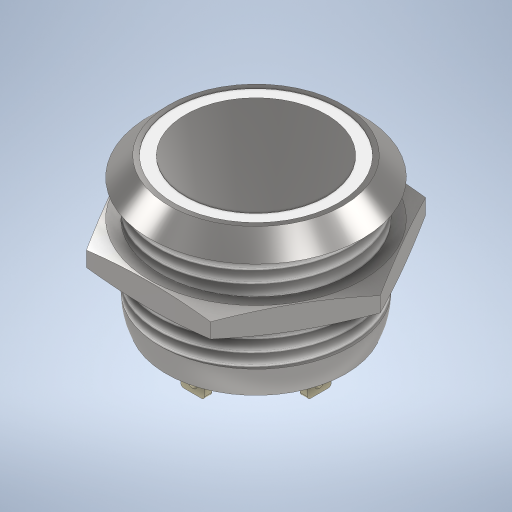
# Autodesk Inventor part: 16mm LED Pushbutton
Saved by Autodesk Inventor 2024 (Build 280153000, 153)
## iProperties
Created: 2024-08-19
Part Number: 16mm LED Pushbutton
Material: Stainless Steel
Document SubType Name: Modeling
Designer: Ishaan
Density: 8 g/cm^3
Appearance: Semi-Polished
Author: Ishaan
Autodesk Inventor part; units mm, degrees
ref_plane "YZ Plane" through (0, 0, 0) normal (1, 0, 0) x (0, 1, 0)
sketch "Sketch1" plane through (0, 0, 0) normal (0, 0, 1) x (1, 0, 0)
  line L0 (0, 11.85) -> (7.3, 11.85)
  line L1 (7.3, 11.85) -> (8.9, 10.25)
  line L2 (8.9, 10.25) -> (8, 10.25)
  line L3 (8, 10.25) -> (8, 2)
  arc A0 (7.5, -0.25) -> (8, 2) centre (2.6875, 2) ccw
  line L4 (7.5, -0.25) -> (7.5, 0)
  line L5 (7.5, 0) -> (0, 0)
  line L6 (0, 0) -> (0, 11.85)
  point P0 (8.45, 10.25)
  dimension "d0" = 8
  dimension "d1" = 1.6
  dimension "d2" = 135
  dimension "d3" = 8.9
  dimension "d5" = 0.25
  dimension "d6" = 0.5
  dimension "d7" = 2
  dimension "d13" = 10.5
  constraints: 14 end point, 3 perpendicular, 2 point on circle, 1 centre point, 1 horizontal, 1 midpoint, 1 parallel, 1 tangent, 1 vertical
  measures "d0" distance between parallel lines of L6 L3
  measures "d1" distance between parallel lines of L0 L2
  measures "d2" angle of L1 L0
  measures "d3" distance from line of L1.end L6
  measures "d5" distance of L4.start L4.end
  measures "d6" distance between parallel lines of L4 L3
  measures "d7" vertical distance of L3.end L5.end
  measures "d13" vertical distance of point (8.45, 10.25) L4.start
revolve "Revolution1" add sketch "Sketch1" angle 360 about axis through (0, 0, 0) along (0, 1, 0)
sketch "Sketch2" plane through (0, 11.85, 0) normal (0, 1, 0) x (1, 0, 0)
  circle A0 centre (0, 0) radius 5.9
  circle A1 centre (0, 0) radius 6.9
  point P0 (0, 0)
  dimension "d9" = 11.8
  dimension "d10" = 1
  constraints: 2 centre point, 1 coincident
  measures "d9" diameter of A0
  measures "d10" radial gap between concentric circles of A0 A1
extrude "Extrusion1" cut sketch "Sketch2" against normal blind 0.05
ref_plane "Work Plane1" through (0, -2.75, 0) normal (0, -1, 0) x (1, 0, 0)
sketch "Sketch3" plane through (0, 0, 0) normal (0, -1, 0) x (1, 0, 0)
  line L0 (-1, 4.7) -> (1, 4.7)
  line L1 (1, 4.7) -> (1, 5.3)
  line L2 (1, 5.3) -> (-1, 5.3)
  line L3 (-1, 5.3) -> (-1, 4.7)
  line L4 (-1, 4.7) -> (1, 5.3) construction
  line L5 (1, 4.7) -> (-1, 5.3) construction
  point P0 (0, 0)
  point P1 (0, 5)
  dimension "d15" = 2
  dimension "d16" = 0.6
  dimension "d17" = 5
  constraints: 12 end point, 2 midpoint, 2 parallel, 1 horizontal, 1 perpendicular, 1 vertical alignment
  measures "d15" distance of L2.end L1.end
  measures "d16" distance of L1.end L0.end
  measures "d17" distance of point (0, 0) point (0, 5)
extrude "Extrusion2" add sketch "Sketch3" along normal up to surface (2.75 mm away)
fillet "Fillet1" radius 0.25 2 edges at (1, -2.75, 5) (-1, -2.75, 5)
sketch "Sketch4" plane through (-1, 0, 5.3) normal (0, 0, 1) x (1, 0, 0)
  arc A0 (0, -2.5) -> (0.25, -2.75) centre (0.25, -2.5) ccw projected
  line L0 (0.25, -2.75) -> (1.75, -2.75) projected
  arc A1 (1.75, -2.75) -> (2, -2.5) centre (1.75, -2.5) ccw projected
  line L1 (2, 0) -> (2, -2.5) projected
  line L2 (0, 0) -> (2, 0) projected
  line L3 (0, 0) -> (0, -2.5) projected
  line L4 (1, -1.5) -> (1, -2) construction
  line L5 (0.6, -1.5) -> (0.6, -2)
  line L6 (1.4, -2) -> (1.4, -1.5)
  arc A2 (1.4, -1.5) -> (0.6, -1.5) centre (1, -1.5) ccw
  arc A3 (0.6, -2) -> (1.4, -2) centre (1, -2) ccw
  point P0 (1, 0)
  point P1 (1, -1.75)
  point P2 (1, -2.75)
  dimension "d21" = 0.8
  dimension "d22" = 0.75
  dimension "d23" = 0.5
  constraints: 8 end point, 4 point on circle, 4 tangent, 2 centre point, 2 midpoint, 1 parallel, 1 vertical, 1 vertical alignment
  measures "d21" diameter of A3
  measures "d22" distance from line of L0 L4.end
  measures "d23" distance of L4.start L4.end
extrude "Extrusion3" cut sketch "Sketch4" against normal up to next contours A2 L6 A3 L5
pattern_circular "Circular Pattern1" count 4 over 360 about axis through (0, 6.125, 0) along (0, 1, 0) of "Extrusion2", "Fillet1", "Extrusion3"
thread "Thread1" size "M16x1" class "6g" standard "ANSI Metric M Profile" length 10
ref_plane "Work Plane2" through (0, 7.25, 0) normal (0, -1, 0) x (1, 0, 0)
sketch "Sketch5" plane through (0, 7.25, 0) normal (0, -1, 0) x (1, 0, 0)
  circle A0 centre (0, 0) radius 8 projected
  circle A1 centre (0, 0) radius 10.9
  line L0 (5.1962, -9) -> (-5.1962, -9)
  line L1 (-5.1962, -9) -> (-10.3923, 0)
  line L2 (-10.3923, 0) -> (-5.1962, 9)
  line L3 (-5.1962, 9) -> (5.1962, 9)
  line L4 (5.1962, 9) -> (10.3923, 0)
  line L5 (10.3923, 0) -> (5.1962, -9)
  point P0 (0, 0)
  point P1 (-5.5552, -9.3782)
  point P2 (-10.8993, -0.1218)
  point P3 (-10.8993, 0.1218)
  point P4 (-5.5552, 9.3782)
  point P5 (-5.3442, 9.5)
  point P6 (5.3442, 9.5)
  point P7 (5.5552, 9.3782)
  point P8 (10.8993, 0.1218)
  point P9 (10.8993, -0.1218)
  point P10 (5.5552, -9.3782)
  point P11 (5.3442, -9.5)
  point P12 (-5.3442, -9.5)
  dimension "d32" = 21.8
  dimension "d33" = 18
  constraints: 12 end point, 2 coincident, 1 centre point, 1 horizontal, 13 other
  measures "d32" diameter of A1
  measures "d33" distance between parallel lines of L3 L0
extrude "Extrusion4" add sketch "Sketch5" along normal blind 2 separate body contours A1 | L0 L1 L2 L3 L4 L5
chamfer "Chamfer1" distance 0.5 distance2 2 1 edges at (-10.9, 7.25, 0) measured on face at (-10.9, 6.75, 0)
chamfer "Chamfer2" distance 0.5 distance2 2 1 edges at (-10.9, 5.25, 0) measured on face at (-10.9, 5.75, 0)
extrude "Extrusion5" cut sketch "Sketch5" along normal through all contours A1 bodies 2
body "Solid1"
